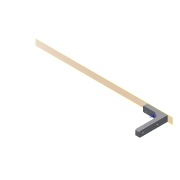
# Autodesk Inventor part: Delivery bin right angle connector
Saved by Autodesk Inventor 2018 (Build 220112000, 112)
## iProperties
Created: 2019-01-05
Part Number: Delivery bin right angle connector
Material: Generic
Document SubType Name: Modeling
Designer: ball
Density: 1 g/cm^3
Appearance: Default
Author: ball
Autodesk Inventor part; units mm, degrees
ref_plane "YZ Plane" through (0, 0, 0) normal (1, 0, 0) x (0, 1, 0)
ref_plane "XZ Plane" through (0, 0, 0) normal (0, 1, 0) x (-1, 0, 0)
ref_plane "XY Plane" through (0, 0, 0) normal (0, 0, 1) x (1, 0, 0)
ref_plane "Work Plane1" through (0, 0, 0) normal (0, 0, 1) x (1, 0, 0)
sketch "Sketch1" plane through (0, 0, 0) normal (0, 0, 1) x (1, 0, 0)
  line L0 (0, 14.859) -> (-322.453, 14.859) construction
  line L1 (-0.635, 0) -> (-321.818, 0) construction
  line L2 (0, 14.859) -> (0, 0.635) construction
  line L3 (2.54, 14.859) -> (2.54, 0)
  line L4 (2.54, 14.859) -> (17.399, 14.859) construction
  line L5 (2.54, 0) -> (-51.4985, 0)
  line L6 (2.54, 14.859) -> (-30.6705, 14.859) construction
  circle A0 centre (-4.7625, 4.7625) radius 1.778 construction
  line L7 (-7.62, 0) -> (-7.62, 14.859) construction
  circle A1 centre (-24.3205, 4.7625) radius 1.778 construction
  circle A2 centre (-43.8785, 4.7625) radius 1.778 construction
  circle A3 centre (-24.3205, 4.7625) radius 1.9685
  circle A4 centre (-43.8785, 4.7625) radius 1.9685
  line L8 (-51.4985, 0) -> (-51.4985, 14.859)
  circle A5 centre (-24.3205, 4.7625) radius 4.8768 construction
  circle A6 centre (-43.8785, 4.7625) radius 4.8768 construction
  line L9 (2.54, 14.859) -> (-51.4985, 14.859)
  point P0 (0, 0)
  dimension "d1" = 2.54
  dimension "d7" = 10.16
  dimension "d9" = 3.937
  dimension "d10" = 3.937
  dimension "d11" = 7.62
  dimension "d12" = 9.7536
  dimension "d13" = 9.7536
  constraints: 20 end point, 7 centre point, 6 point on line, 4 coincident, 4 horizontal, 3 perpendicular, 2 collinear, 1 parallel, 1 vertical, 11 other
  measures "d1" distance between parallel lines of L2 L3
  measures "d7" distance between parallel lines of L7 L3
  measures "d9" diameter of A3
  measures "d10" diameter of A4
  measures "d11" distance from line of L8 A2.centre
  measures "d12" diameter of A5
  measures "d13" diameter of A6
extrude "Extrusion1" add sketch "Sketch1" along normal blind 10.16
sketch "Sketch2" plane through (0, 0, 10.16) normal (0, 0, 1) x (1, 0, 0)
  circle A0 centre (-24.3205, 4.7625) radius 1.9685 construction
  circle A1 centre (-43.8785, 4.7625) radius 1.9685 construction
  line L0 (2.54, 0) -> (2.54, 14.859) projected
  line L1 (2.54, 14.859) -> (-51.4985, 14.859) projected
  line L2 (2.54, 0) -> (-7.62, 0)
  line L3 (-7.62, 0) -> (-7.62, 14.859)
  line L4 (-7.62, 14.859) -> (2.54, 14.859)
  line L5 (2.54, 14.859) -> (2.54, 0)
  point P0 (0, 0)
  dimension "d18" = 10.16
  constraints: 8 end point, 2 parallel, 1 horizontal, 1 perpendicular, 1 point on line
  measures "d18" distance of L3.end L4.end
extrude "Extrusion2" add sketch "Sketch2" along normal blind 63.5
sketch "Sketch3" plane through (-51.4985, 0, 0) normal (0, -1, 0) x (1, 0, 0)
  line L0 (0, 10.16) -> (43.8785, 10.16) projected
  line L1 (43.8785, 10.16) -> (43.8785, 21.59)
  line L2 (43.8785, 10.16) -> (43.8785, 73.66) projected
  line L3 (43.8785, 10.16) -> (32.4485, 10.16)
  line L4 (32.4485, 10.16) -> (43.8785, 21.59)
  point P0 (51.4985, 0)
  dimension "d21" = 11.43
  dimension "d22" = 11.43
  constraints: 6 end point, 2 point on line
  measures "d21" distance of L0.end L1.end
  measures "d22" distance of L0.end L3.end
extrude "Extrusion3" add sketch "Sketch3" against normal blind 14.859
sketch "Sketch4" plane through (0, 0, 10.16) normal (0, 0, 1) x (1, 0, 0)
  circle A0 centre (-24.3205, 4.7625) radius 1.9685 construction
  circle A1 centre (-24.3205, 4.7625) radius 4.8768 construction
  point P0 (0, 0)
  dimension "d25" = 9.7536
  constraints: 1 centre point, 1 coincident
  measures "d25" diameter of A1
sketch "Sketch5" plane through (-7.62, 0, 73.66) normal (-1, 0, 0) x (0, 0, 1)
  line L0 (0, 7.4295) -> (-52.07, 7.4295) construction
  line L1 (-52.07, 14.859) -> (-52.07, 0) construction
  line L2 (-52.07, 14.859) -> (0, 14.859) construction
  circle A0 centre (-46.99, 7.4295) radius 1.9685
  circle A1 centre (-10.16, 7.4295) radius 1.9685
  line L3 (-73.66, 0) -> (-73.66, 14.859) projected
  dimension "d26" = 7.4295
  dimension "d27" = 3.937
  dimension "d28" = 5.08
  dimension "d29" = 3.937
  dimension "d30" = 63.5
  constraints: 2 centre point, 2 end point, 2 point on line, 1 horizontal, 1 midpoint
  measures "d26" distance between parallel lines of L2 L0
  measures "d27" diameter of A0
  measures "d28" distance of L0.end A0.centre
  measures "d29" diameter of A1
  measures "d30" distance from line of A1.centre L3
extrude "Extrusion4" cut sketch "Sketch5" against normal through all
fillet "Fillet1" radius 3.175 4 edges at (-2.54, 14.859, 73.66) (-51.4985, 0, 5.08) (-51.4985, 14.859, 5.08) (-2.54, 0, 73.66)
body "Solid1"
